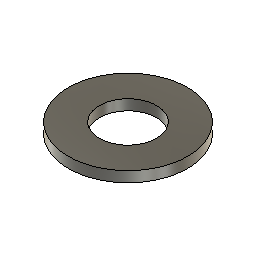
Small Washer, 0.03125 (Steel) v2 (Autodesk Fusion 360 design; units mm, degrees)
Autodesk Fusion 360 part; units mm, degrees
sketch "Sketch1" plane through (0, 0, 0) normal (0, 0, 1) x (1, 0, 0)
  circle A0 centre (0, 0) radius 2.1463
  circle A1 centre (0, 0) radius 4.4958
  dimension "d1" = 4.2926
  dimension "d2" = 8.9916
  constraint coincident A0.centre A1.centre
  constraint concentric A0 A1
  measures "d1" diameter of A0
  measures "d2" diameter of A1
extrude "Extrude1" add sketch "Sketch1" along normal blind 0.7937
equation "d3 = ( 1 / 32 ) * 1 in"
